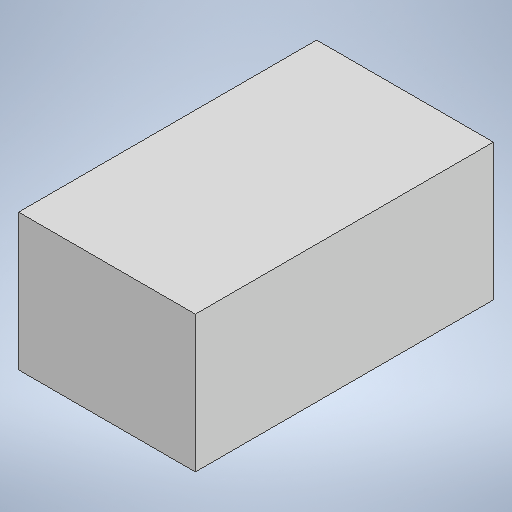
# Autodesk Inventor part: prop
Saved by Autodesk Inventor 2025.2 (Build 292293000, 293)
## iProperties
Created: 2025-03-25
Part Number: prop
Material: Všeobecné
Document SubType Name: Modeling
Designer: hepma_axt67em
Density: 1 g/cm^3
Appearance: Výchozí
Author: hepma_axt67em
Autodesk Inventor part; units mm, degrees
ref_plane "YZ Plane" through (0, 0, 0) normal (1, 0, 0) x (0, 1, 0)
ref_plane "XZ Plane" through (0, 0, 0) normal (0, 1, 0) x (-1, 0, 0)
ref_plane "XY Plane" through (0, 0, 0) normal (0, 0, 1) x (1, 0, 0)
sketch "Náčrt1" plane through (0, 0, 0) normal (0, 0, 1) x (1, 0, 0)
  line L0 (0, 0) -> (5.9308, 0)
  line L1 (5.9308, 0) -> (5.9308, 4.5851)
  line L2 (5.9308, 4.5851) -> (0, 4.5851)
  line L3 (0, 4.5851) -> (0, 0)
  constraints: 8 end point, 2 parallel, 1 horizontal, 1 perpendicular
extrude "Vysunutí1" add sketch "Náčrt1" along normal blind 10
